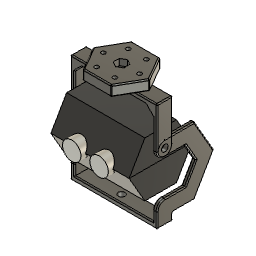
polychrome-sensor-box (Autodesk Fusion 360 design; units mm, degrees)
Autodesk Fusion 360 part; units mm, degrees
note: some values were not read from the file. Set by a fixed rule: which face or edge a step refers to.
(part 1 of 2)
sketch "base" plane through (0, 0, 0) normal (0, 0, 1) x (1, 0, 0) in component "Component"
  line L0 (31.5, 19.5) -> (-31.5, 19.5)
  line L1 (-31.5, 19.5) -> (-31.5, -19.5)
  line L2 (-31.5, -19.5) -> (31.5, -19.5)
  line L3 (31.5, -19.5) -> (31.5, 19.5)
  line L4 (31.5, 19.5) -> (-31.5, -19.5) construction
  line L5 (-31.5, 19.5) -> (31.5, -19.5) construction
  dimension "d5" = 63
  dimension "d6" = 39
  constraint horizontal L0
  constraint perpendicular L0 L1
  constraint parallel L0 L2
  constraint parallel L1 L3
  constraint coincident L4 origin
  constraint coincident L5 origin
  measures "d5" distance of L1.end L2.end
  measures "d6" distance of L0.end L1.end
extrude "Extrude1" add sketch "base" along normal blind 36 makes body 1 in component "Component"
shell "Shell1" thickness 2 removed faces 1 at (10.5, 6.5, 36) on bodies 1 in component "Component"
sketch "sensors" plane through (0, -19.5, 0) normal (0, -1, 0) x (1, 0, 0) in component "Component"
  line L0 (-31.5, 0) -> (31.5, 0)
  line L1 (31.5, 0) -> (31.5, 36)
  line L2 (31.5, 36) -> (-31.5, 36)
  line L3 (-31.5, 36) -> (-31.5, 0)
  line L4 (-31.5, 24.25) -> (31.5, 24.25) construction
  line L5 (0, 36) -> (0, 0) construction
  line L6 (6.219, 36) -> (6.219, 0) construction
  circle A0 centre (18.719, 24.25) radius 8.65
  circle A1 centre (-6.281, 24.25) radius 8.65
  dimension "d10" = 24.25
  dimension "d63" = 6.219
  dimension "d64" = 17.3
  dimension "d65" = 12.5
  constraint coincident L3 L4.start
  constraint coincident L1 L4.end
  constraint perpendicular L1 L4
  constraint midpoint L2 L5.start
  constraint coincident L5.end origin
  constraint coincident L2 L6.start
  constraint coincident L0 L6.end
  constraint perpendicular L0 L6
  constraint coincident L4 A0.centre
  constraint symmetric L6 A0 A1
  measures "d10" distance of L0 L4
  measures "d63" distance of L5 L6
  measures "d64" diameter of A0
  measures "d65" distance of L6 A0.centre
extrude "Extrude2" cut sketch "sensors" against normal up to surface (2 mm away) contours A0 | A1 bodies 1 in component "Component"
sketch "rj45" plane through (-31.5, 0, 0) normal (-1, 0, 0) x (0, -1, 0) in component "Component"
  line L0 (-19.5, 0) -> (19.5, 0)
  line L1 (19.5, 0) -> (19.5, 36)
  line L2 (19.5, 36) -> (-19.5, 36)
  line L3 (-19.5, 36) -> (-19.5, 0)
  line L4 (-4.499, 36) -> (-4.499, 0) construction
  line L5 (-19.5, 13.6) -> (19.5, 13.6) construction
  line L6 (3.901, 21) -> (-12.899, 21)
  line L7 (-12.899, 21) -> (-12.899, 6.2)
  line L8 (-12.899, 6.2) -> (3.901, 6.2)
  line L9 (3.901, 6.2) -> (3.901, 21)
  line L10 (3.901, 21) -> (-12.899, 6.2) construction
  line L11 (-12.899, 21) -> (3.901, 6.2) construction
  point P0 (-4.499, 13.6)
  dimension "d57" = 15.001
  dimension "d58" = 13.6
  dimension "d59" = 16.8
  dimension "d60" = 14.8
  constraint coincident L2 L4.start
  constraint coincident L0 L4.end
  constraint perpendicular L0 L4
  constraint coincident L3 L5.start
  constraint coincident L1 L5.end
  constraint perpendicular L1 L5
  constraint horizontal L6
  constraint perpendicular L6 L7
  constraint parallel L6 L8
  constraint parallel L7 L9
  constraint coincident L10 P0
  constraint coincident L11 P0
  constraint coincident L4 P0
  constraint coincident L5 P0
  measures "d57" distance of L3 L4
  measures "d58" distance of L0 L5
  measures "d59" distance of L7.end L8.end
  measures "d60" distance of L6.end L7.end
extrude "Extrude3" cut sketch "rj45" against normal up to surface (2 mm away) contours L6 L7 L8 L9 bodies 1 in component "Component"
sketch "Sketch2" plane through (0, 0, 0) normal (0, 0, 1) x (1, 0, 0) in component "sensor"
  line L0 (0, 0) -> (57, 0)
  line L1 (57, 0) -> (57, 30)
  line L2 (57, 30) -> (0, 30)
  line L3 (0, 30) -> (0, 0)
  dimension "d66" = 57
  dimension "d67" = 30
  constraint horizontal L0
  constraint vertical L1
  constraint horizontal L2
  constraint vertical L3
  constraint coincident L0.start L3.end
  measures "d66" distance of L0.start L0.end
  measures "d67" distance of L0.start L2.end
extrude "Extrude1'" add sketch "Sketch2" along normal blind 1.6 separate body makes body 2 in component "sensor"
sketch "Sketch3" plane through (0, 0, 1.6) normal (0, 0, 1) x (-1, 0, 0) in component "sensor"
  line L0 (0, -30) -> (0, 0)
  line L1 (0, 0) -> (-57, 0)
  line L2 (-57, 0) -> (-57, -30)
  line L3 (-57, -30) -> (0, -30)
  line L4 (-21.823, -25.799) -> (5.277, -25.799)
  line L5 (5.277, -25.799) -> (5.277, -8.999)
  line L6 (5.277, -8.999) -> (-21.823, -8.999)
  line L7 (-21.823, -8.999) -> (-21.823, -25.799)
  line L8 (-21.823, -25.799) -> (5.277, -8.999) construction
  line L9 (5.277, -25.799) -> (-21.823, -8.999) construction
  line L10 (-29.029, -6.623) -> (-40.409, -6.623)
  line L11 (-40.409, -6.623) -> (-40.409, -3.283)
  line L12 (-40.409, -3.283) -> (-29.029, -3.283)
  line L13 (-29.029, -3.283) -> (-29.029, -6.623)
  line L14 (-29.029, -6.623) -> (-40.409, -3.283) construction
  line L15 (-40.409, -6.623) -> (-29.029, -3.283) construction
  point P0 (-8.273, -17.399)
  point P1 (-8.273, -17.399)
  point P2 (-34.719, -4.953)
  point P3 (-34.719, -4.953)
  dimension "d70" = 12.601
  dimension "d71" = 8.273
  dimension "d72" = 27.1
  dimension "d73" = 16.8
  dimension "d76" = 25.047
  dimension "d77" = 34.719
  dimension "d78" = 11.38
  dimension "d79" = 3.34
  constraint horizontal L4
  constraint perpendicular L4 L5
  constraint parallel L4 L6
  constraint parallel L5 L7
  constraint coincident L8 P1
  constraint coincident L9 P1
  constraint coincident P1 P0
  constraint horizontal L10
  constraint perpendicular L10 L11
  constraint parallel L10 L12
  constraint parallel L11 L13
  constraint coincident L14 P3
  constraint coincident L15 P3
  constraint coincident P3 P2
  measures "d70" distance of L3 P1
  measures "d71" distance of L0 P1
  measures "d72" distance of L5.end L6.end
  measures "d73" distance of L4.end L5.end
  measures "d76" distance of L3 P3
  measures "d77" distance of L0 P3
  measures "d78" distance of L11.end L12.end
  measures "d79" distance of L10.end L11.end
extrude "Extrude2'" add sketch "Sketch3" along normal blind 14.8 contours L0 L4 L6 L7 | L0 L4 L5 L6 bodies 2 in component "sensor"
extrude "Extrude3'" add sketch "Sketch3" along normal blind 28.8 contours L10 L11 L12 L13 bodies 2 in component "sensor"
sketch "Sketch4" plane through (0, 3.283, 0) normal (0, -1, 0) x (1, 0, 0) in component "sensor"
  line L0 (29.029, 1.6) -> (40.409, 1.6)
  line L1 (40.409, 1.6) -> (40.409, 30.4)
  line L2 (40.409, 30.4) -> (29.029, 30.4)
  line L3 (29.029, 30.4) -> (29.029, 1.6)
  line L4 (29.029, 30.4) -> (40.2114, 30.4)
  line L5 (40.2114, 30.4) -> (40.2114, 9.1)
  line L6 (40.2114, 9.1) -> (29.029, 9.1)
  line L7 (29.029, 9.1) -> (29.029, 30.4)
  dimension "d82" = 21.3
  constraint horizontal L4
  constraint vertical L5
  constraint horizontal L6
  constraint vertical L7
  constraint coincident L2.end L3.start
  measures "d82" distance of L2.end L6.end
extrude "Extrude4" add sketch "Sketch4" along normal blind 8 separate body contours L2 L3 L4 L5 L6 L7 makes body 3 in component "sensor"
ref_plane "WorkPlane1" through (34.6202, -0.717, 19.75) normal (1, 0, 0) x (0, 0, 1) in component "sensor"
ref_plane "WorkPlane2" through (57.7702, -0.717, 19.75) normal (1, 0, 0) x (0, 0, 1) in component "sensor"
ref_plane "WorkPlane3" through (11.4702, -0.717, 19.75) normal (1, 0, 0) x (0, 0, 1) in component "sensor"
extrude "Extrude5" add 1 faces at (40.2114, -2.0503, 16.2) along direction (1, 0, 0) up to surface (17.5588 mm away) and the other way up to surface (28.7412 mm away) on bodies 3 bodies 2 3 in component "sensor"
sketch "Sketch5" plane through (0, -4.717, 0) normal (0, -1, 0) x (1, 0, 0) in component "sensor"
  line L0 (11.4702, 9.1) -> (57.7702, 9.1)
  line L1 (57.7702, 9.1) -> (57.7702, 30.4)
  line L2 (57.7702, 30.4) -> (11.4702, 30.4)
  line L3 (11.4702, 30.4) -> (11.4702, 9.1)
  line L4 (11.4702, 19.75) -> (57.7702, 19.75) construction
  line L5 (34.6202, 30.4) -> (34.6202, 9.1) construction
  circle A0 centre (21.4702, 19.75) radius 8.9
  circle A1 centre (47.7702, 19.75) radius 8.9
  dimension "d91" = 17.8
  dimension "d92" = 10
  constraint midpoint L3 L4.start
  constraint midpoint L1 L4.end
  constraint midpoint L2 L5.start
  constraint midpoint L0 L5.end
  constraint coincident L4 A0.centre
  constraint symmetric L5 A0 A1
  measures "d91" diameter of A0
  measures "d92" distance of L4.start A0.centre
extrude "Extrude6" add sketch "Sketch5" along normal blind 15 contours A0 | A1 bodies 2 in component "sensor"
sketch "Sketch2 (2)" plane through (56.4993, 0, 0) normal (1, 0, 0) x (0, 1, 0) in component "Component'"
  line L0 (-8.1168, 6.6878) -> (-0.1168, 6.6878)
  line L1 (-0.1168, 6.6878) -> (-0.1168, 27.9878)
  line L2 (-0.1168, 27.9878) -> (-8.1168, 27.9878)
  line L3 (-8.1168, 27.9878) -> (-8.1168, 6.6878)
  line L4 (-8.1168, 27.9878) -> (26.6636, -2.3727) construction
  line L5 (-8.8786, 28.508) -> (-13.3996, 4.9377)
  line L6 (-13.3996, 4.9377) -> (4.7524, -10.7628)
  line L7 (4.7524, -10.7628) -> (27.4254, -2.893)
  line L8 (27.4254, -2.893) -> (31.9464, 20.6774)
  line L9 (31.9464, 20.6774) -> (13.7944, 36.3779)
  line L10 (13.7944, 36.3779) -> (-8.8786, 28.508)
  line L11 (-15.5813, 4.1804) -> (4.3173, -13.0308)
  line L12 (4.3173, -13.0308) -> (29.1721, -4.4037)
  line L13 (29.1721, -4.4037) -> (34.1281, 21.4346)
  line L14 (34.1281, 21.4346) -> (14.2295, 38.6459)
  line L15 (14.2295, 38.6459) -> (-10.6253, 30.0188)
  line L16 (-10.6253, 30.0188) -> (-15.5813, 4.1804)
  point P0 (9.2734, 12.8075)
  dimension "d96" = 24
  dimension "d104" = 2
  constraint coincident L2.end L3.start
  constraint midpoint L4 P0
  measures "d96" distance of L5.start P0
ref_plane "WorkPlane4" through (34.6202, 0.953, 19.75) normal (0, 0, 1) x (1, 0, 0) in component "sensor"
sketch "Sketch3 (2)" plane through (56.4993, 0, 0) normal (1, 0, 0) x (0, 1, 0) in component "Component'"
  line L0 (38.5849, 17.0433) -> (25.1323, 40.4534)
  line L1 (25.1323, 40.4534) -> (-1.8676, 40.5081)
  line L2 (-1.8676, 40.5081) -> (-15.415, 17.1529)
  line L3 (-15.415, 17.1529) -> (-1.9625, -6.2572)
  line L4 (-1.9625, -6.2572) -> (25.0375, -6.3119)
  line L5 (25.0375, -6.3119) -> (38.5849, 17.0433)
  line L6 (-3.1212, -8.2548) -> (26.1881, -8.3143)
  line L7 (26.1881, -8.3143) -> (40.8943, 17.0387)
  line L8 (40.8943, 17.0387) -> (26.2911, 42.451)
  line L9 (26.2911, 42.451) -> (-3.0183, 42.5105)
  line L10 (-3.0183, 42.5105) -> (-17.7244, 17.1576)
  line L11 (-17.7244, 17.1576) -> (-3.1212, -8.2548)
  point P0 (11.5849, 17.0981)
  dimension "d111" = 27
  dimension "d112" = 2
  measures "d111" distance of L0.start P0
sketch "inner base" plane through (0, 0, 2) normal (0, 0, 1) x (-1, 0, 0) in component "Component"
  line L0 (-29.5, 17.5) -> (-29.5, -17.5)
  line L1 (-29.5, -17.5) -> (29.5, -17.5)
  line L2 (29.5, -17.5) -> (29.5, 17.5)
  line L3 (29.5, 17.5) -> (-29.5, 17.5)
  line L4 (29.5, -17.5) -> (9.5, -17.5)
  line L5 (9.5, -17.5) -> (9.5, -14)
  line L6 (9.5, -14) -> (29.5, -14)
  line L7 (29.5, -14) -> (29.5, -17.5)
  line L8 (29.5, -17.5) -> (26, -17.5)
  line L9 (26, -17.5) -> (26, 5.9)
  line L10 (26, 5.9) -> (29.5, 5.9)
  line L11 (29.5, 5.9) -> (29.5, -17.5)
  line L12 (-29.5, -17.5) -> (-29.5, 17.5) construction
  line L13 (26.5811, 12.7) -> (-29.5, 12.7) construction
  line L14 (-29.5, -17.5) -> (-19.5, -17.5)
  line L15 (-19.5, -17.5) -> (-19.5, 17.5)
  line L16 (-19.5, 17.5) -> (-29.5, 17.5)
  line L17 (-29.5, 17.5) -> (-29.5, -17.5)
  line L18 (29.5, 5.9) -> (19.5, 5.9)
  line L19 (19.5, 5.9) -> (19.5, 17.5)
  line L20 (19.5, 17.5) -> (29.5, 17.5)
  line L21 (29.5, 17.5) -> (29.5, 5.9)
  dimension "d31" = 20
  dimension "d32" = 3.5
  dimension "d33" = 3.5
  dimension "d34" = 23.4
  dimension "d36" = 7.4
  dimension "d37" = 59
  dimension "d38" = 10
  dimension "d40" = 10
  constraint horizontal L4
  constraint vertical L5
  constraint horizontal L6
  constraint vertical L7
  constraint coincident L1.end L2.start
  constraint horizontal L8
  constraint vertical L9
  constraint horizontal L10
  constraint vertical L11
  constraint coincident L1 L0.end
  constraint coincident L3 L0.start
  constraint perpendicular L3 L12
  constraint coincident L12 L13.end
  constraint perpendicular L12 L13
  constraint horizontal L14
  constraint vertical L15
  constraint horizontal L16
  constraint vertical L17
  constraint horizontal L18
  constraint vertical L19
  constraint horizontal L20
  constraint vertical L21
  measures "d31" distance of L1.end L4.end
  measures "d32" distance of L1.end L6.end
  measures "d33" distance of L1.end L8.end
  measures "d34" distance of L1.end L10.end
  measures "d36" distance of L10.end L13.start
  measures "d37" distance of L2 L12
  measures "d38" distance of L0.end L14.end
  measures "d40" distance of L10.end L18.end
extrude "Extrude4'" add sketch "inner base" along normal blind 3 contours L0 L1 L3 L14 L15 L16 L17 | L2 L3 L10 L18 L19 L20 L21 | L1 L4 L5 L6 L9 | L1 L2 L4 L6 L7 L8 L9 L11 | L2 L6 L9 L10 L11 L18 bodies 1 in component "Component"
sketch "board holes" plane through (0, 0, 5) normal (0, 0, 1) x (-1, 0, 0) in component "Component"
  line L0 (29.5, 17.5) -> (19.5, 17.5)
  line L1 (19.5, 17.5) -> (19.5, 5.9)
  line L2 (19.5, 5.9) -> (26, 5.9)
  line L3 (26, 5.9) -> (26, -14)
  line L4 (26, -14) -> (9.5, -14)
  line L5 (9.5, -14) -> (9.5, -17.5)
  line L6 (9.5, -17.5) -> (29.5, -17.5)
  line L7 (29.5, -17.5) -> (29.5, 17.5)
  line L8 (29.1, -17.1) -> (-27.9, -17.1) construction
  line L9 (-27.9, -17.1) -> (-27.9, 12.9) construction
  line L10 (-27.9, 12.9) -> (29.1, 12.9) construction
  line L11 (29.1, 12.9) -> (29.1, -17.1) construction
  line L12 (26.893, -17.1) -> (26.893, 12.9) construction
  line L13 (29.1, -15.04) -> (-27.9, -15.04) construction
  line L14 (29.1, 10.614) -> (-27.9, 10.614) construction
  circle A0 centre (26.893, -15.04) radius 1.25
  circle A1 centre (26.893, 10.614) radius 1.25
  line L15 (-25.9, -17.1) -> (-25.9, 12.9) construction
  circle A2 centre (-25.9, -15.04) radius 1.25
  circle A3 centre (-25.9, 10.614) radius 1.25
  dimension "d43" = 57
  dimension "d44" = 30
  dimension "d45" = 0.4
  dimension "d46" = 0.4
  dimension "d47" = 2.207
  dimension "d48" = 2.06
  dimension "d49" = 2.286
  dimension "d50" = 2.5
  dimension "d51" = 2.5
  dimension "d52" = 52.793
  dimension "d53" = 2.5
  dimension "d54" = 2.5
  constraint horizontal L8
  constraint vertical L9
  constraint horizontal L10
  constraint vertical L11
  constraint coincident L8 L12.start
  constraint coincident L10 L12.end
  constraint perpendicular L10 L12
  constraint coincident L11 L13.start
  constraint coincident L9 L13.end
  constraint perpendicular L9 L13
  constraint coincident L11 L14.start
  constraint coincident L9 L14.end
  constraint perpendicular L9 L14
  constraint coincident L12 A0.centre
  constraint coincident L13 A0.centre
  constraint coincident L12 A1.centre
  constraint coincident L14 A1.centre
  constraint coincident L8 L15.start
  constraint coincident L10 L15.end
  constraint perpendicular L10 L15
  constraint coincident L13 A2.centre
  constraint coincident L15 A2.centre
  constraint coincident L14 A3.centre
  constraint coincident L15 A3.centre
  measures "d43" distance of L8.start L8.end
  measures "d44" distance of L8.start L10.end
  measures "d45" distance of L6 L8
  measures "d46" distance of L7 L11
  measures "d47" distance of L11 L12
  measures "d48" distance of L8 L13
  measures "d49" distance of L10 L14
  measures "d50" diameter of A0
  measures "d51" diameter of A1
  measures "d52" distance of L12 L15
  measures "d53" diameter of A2
  measures "d54" diameter of A3
extrude "Extrude5'" cut sketch "board holes" against normal blind 4 draft -8 contours A0 | A1 | A2 | A3 bodies 1 in component "Component"
sketch "Sketch6" plane through (31.5, 0, 0) normal (1, 0, 0) x (0, 1, 0) in component "Component"
  line L0 (-19.5, 0) -> (19.5, 0)
  line L1 (19.5, 0) -> (19.5, 36)
  line L2 (19.5, 36) -> (-19.5, 36)
  line L3 (-19.5, 36) -> (-19.5, 0)
  line L4 (-19.5, 36) -> (19.5, 0) construction
  line L5 (19.5, 36) -> (-19.5, 0) construction
  constraint coincident L2.end L3.start
  constraint coincident L0.end L1.start
  constraint coincident L1.end L2.start
  constraint coincident L0.start L3.end
extrude "Extrude6'" add sketch "Sketch3 (2)" along normal blind 2 separate body contours L0 L1 L2 L3 L4 L5 makes body 4 in component "Component'"
extrude "Extrude7" add sketch "Sketch3 (2)" along normal blind 2 and the other way up to surface (57.7702 mm away) bodies 4 in component "Component'"
sketch "Sketch6 (2)" plane through (0, 0, 0) normal (0, 0, -1) x (1, 0, 0) in component "sensor"
  line L0 (0, 0) -> (0, -30)
  line L1 (0, -30) -> (57, -30)
  line L2 (57, -30) -> (57, 0)
  line L3 (57, 0) -> (0, 0)
  line L4 (0, -2.286) -> (56.7828, -2.286) construction
  line L5 (0, -27.94) -> (57, -27.94) construction
  line L6 (2.207, 0) -> (2.207, -30) construction
  line L7 (55, 0) -> (55, -30) construction
  circle A0 centre (55, -2.4077) radius 1.262
  circle A1 centre (55, -27.94) radius 1.262
  circle A2 centre (2.207, -27.94) radius 1.262
  circle A3 centre (2.207, -2.286) radius 1.262
  line L8 (6.5, 0) -> (47, 0)
  line L9 (47, 0) -> (47, -30)
  line L10 (47, -30) -> (6.5, -30)
  line L11 (6.5, -30) -> (6.5, 0)
  line L12 (47, -10) -> (57, -10)
  line L13 (57, -10) -> (57, -20)
  line L14 (57, -20) -> (47, -20)
  line L15 (47, -20) -> (47, -10)
  line L16 (0, -6.5) -> (6.5, -6.5)
  line L17 (6.5, -6.5) -> (6.5, -27.5)
  line L18 (6.5, -27.5) -> (0, -27.5)
  line L19 (0, -27.5) -> (0, -6.5)
  dimension "d119" = 2.286
  dimension "d120" = 2.207
  dimension "d121" = 2.06
  dimension "d122" = 2
  dimension "d123" = 2.524
  dimension "d124" = 2.524
  dimension "d125" = 2.524
  dimension "d126" = 2.524
  dimension "d131" = 6.5
  dimension "d132" = 10
  dimension "d133" = 10
  dimension "d134" = 10
  dimension "d135" = 6.5
  dimension "d136" = 2.5
  constraint coincident L0 L4.start
  constraint perpendicular L2 L4
  constraint coincident L0 L5.start
  constraint coincident L2 L5.end
  constraint perpendicular L2 L5
  constraint coincident L3 L6.start
  constraint coincident L1 L6.end
  constraint perpendicular L1 L6
  constraint coincident L3 L7.start
  constraint coincident L1 L7.end
  constraint perpendicular L1 L7
  constraint coincident L7 A0.centre
  constraint coincident L5 A1.centre
  constraint coincident L7 A1.centre
  constraint coincident L6 A2.centre
  constraint coincident L5 A2.centre
  constraint coincident L4 A3.centre
  constraint coincident L6 A3.centre
  constraint horizontal L8
  constraint vertical L9
  constraint horizontal L10
  constraint vertical L11
  constraint coincident L1 L9.end
  constraint coincident L3 L8.start
  constraint horizontal L12
  constraint vertical L13
  constraint horizontal L14
  constraint vertical L15
  constraint coincident L2 L13.end
  constraint coincident L9 L12.start
  constraint horizontal L16
  constraint vertical L17
  constraint horizontal L18
  constraint vertical L19
  constraint coincident L11 L17.end
  constraint coincident L0 L16.start
  measures "d119" distance of L3 L4
  measures "d120" distance of L0 L6
  measures "d121" distance of L1 L5
  measures "d122" distance of L2 L7
  measures "d123" diameter of A0
  measures "d124" diameter of A1
  measures "d125" diameter of A2
  measures "d126" diameter of A3
  measures "d131" distance of L0 L11
  measures "d132" distance of L2 L9
  measures "d133" distance of L3 L12
  measures "d134" distance of L1 L14
  measures "d135" distance of L3 L16
  measures "d136" distance of L1 L18
extrude "Extrude7'" add sketch "Sketch6 (2)" along normal blind 2 contours L0 A2 L11 L16 L17 L18 L19 | L1 L3 L8 L9 L10 L11 L15 L17 | A2 L18 | L2 L9 L12 L13 L14 L15 picked at (2.177, -27.2271) bodies 2 in component "sensor"
extrude "Extrude8" add sketch "Sketch6 (2)" along normal blind 4 draft -8 contours A2 L18 | A2 L18 | A0 | A1 | A3 bodies 2 in component "sensor"
ref_plane "WorkPlane5" through (34.6202, -4.717, 19.75) normal (1, 0, 0) x (0, 0, -1) in component "sensor"
ref_plane "WorkPlane4" through (0.8755, 14.3886, 3.4379) normal (-1, 0, 0) x (0, -1, 0) in component "enclosure"
sketch "Sketch3 (3)" plane through (0.8755, 0, 0) normal (-1, 0, 0) x (0, -1, 0) in component "enclosure"
  line L0 (-29.3886, 3.6379) -> (0.6114, 3.6379) construction
  line L1 (5.3284, 34.0379) -> (5.3284, 12.7379) construction
  line L2 (5.3284, 23.3879) -> (-27.8442, 23.3879) construction
  line L3 (-14.3886, 3.6379) -> (-14.3886, 31.9391) construction
  line L4 (-0.3886, -0.8608) -> (13.6114, 23.3879)
  line L5 (13.6114, 23.3879) -> (-0.3886, 47.6367)
  line L6 (-0.3886, 47.6367) -> (-28.3886, 47.6367)
  line L7 (-28.3886, 47.6367) -> (-42.3886, 23.3879)
  line L8 (-42.3886, 23.3879) -> (-28.3886, -0.8608)
  line L9 (-28.3886, -0.8608) -> (-0.3886, -0.8608)
  line L10 (-5.8886, 1.6379) -> (-26.8886, 1.6379)
  line L11 (-44.698, 23.3879) -> (-29.5433, -2.8608)
  line L12 (-29.5433, -2.8608) -> (0.7661, -2.8608)
  line L13 (0.7661, -2.8608) -> (15.9208, 23.3879)
  line L14 (15.9208, 23.3879) -> (0.7661, 49.6367)
  line L15 (0.7661, 49.6367) -> (-29.5433, 49.6367)
  line L16 (-29.5433, 49.6367) -> (-44.698, 23.3879)
  point P0 (5.3284, 34.0379)
  point P1 (5.3284, 12.7379)
  point P2 (0.6114, 3.6379)
  point P3 (-29.3886, 3.6379)
  point P4 (-14.3886, 23.3879)
  dimension "d156" = 28
  dimension "d157" = 2
  constraint coincident P3 L0.start
  constraint coincident P2 L0.end
  constraint coincident P0 L1.start
  constraint coincident P1 L1.end
  constraint midpoint L1 L2.start
  constraint perpendicular L1 L2
  constraint midpoint L0 L3.start
  constraint perpendicular L0 L3
  constraint coincident L2 P4
  constraint coincident L3 P4
  constraint parallel L9 L10
  measures "d156" distance of L4.start P4
extrude "Extrude4''" add sketch "Sketch3 (3)" along normal blind 2 separate body contours L4 L5 L6 L7 L8 L9 makes body 5 in component "enclosure"
mirror "Mirror1" about plane through (36.4957, -5.3284, 23.3879) normal (1, 0, 0) of bodies 5 makes body 6 in component "enclosure"
extrude "Extrude5''" add sketch "Sketch3 (3)" along normal blind 2 and the other way up to surface (73.2404 mm away) separate body makes body 7 in component "enclosure"
extrude "Extrude6''" add 1 faces at (49.0357, 19.0552, -0.8608) along direction (0, 0, 1) up to surface (4.4987 mm away) on bodies 7 bodies 7 in component "enclosure"
extrude "Extrude7''" add 1 faces at (49.0357, 0.3886, 2.1384) along direction (0, -1, 0) up to surface end surface through (0.8755, 0.3886, -0.8608) normal (0, 0.866025, 0.5) offset 0 on bodies 7 bodies 7 in component "enclosure"
extrude "Extrude8'" add 1 faces at (23.9556, 28.3886, 0.6388) along direction (0, 1, 0) up to surface end surface through (0.8755, 42.3886, 23.3879) normal (0, -0.866025, 0.5) offset 0 on bodies 7 bodies 7 in component "enclosure"
ref_plane "WorkPlane5" through (36.4957, 14.3886, 23.3879) normal (0, 0, 1) x (0, 1, 0) in component "enclosure"
split "Split1" by plane through (36.4957, 14.3886, 23.3879) normal (0, 0, 1) bodies 7 makes body 8 at (49.0357, -10.8693, 32.1375) in component "enclosure"
sketch "Sketch4 (2)" plane through (-1.1245, 0, 0) normal (-1, 0, 0) x (0, -1, 0) in component "enclosure"
  line L0 (15.9208, 23.3879) -> (13.6114, 23.3879)
  line L1 (13.6114, 23.3879) -> (2.2088, 3.6379)
  line L2 (2.2088, 3.6379) -> (-30.9859, 3.6379)
  line L3 (-30.9859, 3.6379) -> (-42.3886, 23.3879)
  line L4 (-42.3886, 23.3879) -> (-44.698, 23.3879)
  line L5 (-44.698, 23.3879) -> (-29.5433, -2.8608)
  line L6 (-29.5433, -2.8608) -> (0.7661, -2.8608)
  line L7 (0.7661, -2.8608) -> (15.9208, 23.3879)
  line L8 (13.6114, 23.3879) -> (11.6114, 23.3879)
  line L9 (11.6114, 23.3879) -> (9.6114, 19.9238)
  line L10 (9.6114, 19.9238) -> (11.1114, 19.0578)
  line L11 (9.6114, 16.4597) -> (6.1473, 18.4597) construction
  line L12 (6.1473, 18.4597) -> (11.302, 27.3879)
  line L13 (-0.3886, 47.6367) -> (13.6114, 23.3879)
  line L14 (8.9188, 19.1242) -> (11.9006, 24.2889) construction
  line L15 (13.0993, 17.6792) -> (7.5473, 20.8846) construction
  line L16 (9.3382, 19.8506) -> (11.0114, 18.8846)
  line L17 (11.6114, 23.3879) -> (10.186, 23.3879) construction
  line L18 (9.3382, 19.8506) -> (11.3805, 23.3879)
  line L19 (11.6114, 23.3879) -> (11.3805, 23.3879)
  line L20 (7.5473, 20.8846) -> (7.5473, 11.8372) construction
  line L21 (7.5473, 20.8846) -> (7.5473, 12.8846)
  dimension "d172" = 2
  dimension "d173" = 4
  dimension "d174" = 3
  dimension "d175" = 4
  dimension "d177" = 0.2
  dimension "d178" = 0.2
  constraint coincident L0.end L1.start
  constraint parallel L0 L8
  constraint parallel L1 L9
  constraint coincident L1 L10.end
  constraint perpendicular L1 L10
  constraint coincident L1 L11.start
  constraint parallel L10 L11
  constraint coincident L11 L12.start
  constraint coincident L12.end L13
  constraint parallel L9 L12
  constraint parallel L9 L14
  constraint parallel L10 L15
  constraint coincident L15 L16.start
  constraint coincident L14 L16.start
  constraint coincident L15 L16.end
  constraint coincident L1 L16.end
  constraint parallel L8 L17
  constraint coincident L14 L18.end
  constraint coincident L17 L18.end
  constraint perpendicular L2 L20
  constraint coincident L12 L15.end
  constraint coincident L15.end L20
  constraint coincident L15.end L20.start
  constraint coincident L1 L21.end
  constraint coincident L20 L21.end
  constraint coincident L11.end L12.start
  measures "d172" distance of L0.end L8.end
  measures "d173" distance of L8.end L9.end
  measures "d174" distance of L10.end L11.start
  measures "d175" distance of L11.start L11.end
  measures "d177" distance of L9 L14
  measures "d178" distance of L10 L15
extrude "Extrude9" add sketch "Sketch4 (2)" against normal blind 14.4 separate body contours L1 L8 L9 L10 makes body 9 in component "enclosure"
extrude "Extrude10" cut 1 faces at (-1.1245, -12.1114, 21.9446) along direction (1, 0, 0) blind 5.4 on bodies 9 bodies 9 in component "enclosure"
mirror "Mirror2" about plane through (36.4957, -5.3284, 23.3879) normal (1, 0, 0) of bodies 9 makes body 10 in component "enclosure"
extrude "Extrude11" add sketch "Sketch4 (2)" against normal blind 14.4 separate body contours L1 L8 L12 L13 L16 L18 L19 L21 makes body 11 in component "enclosure"
extrude "Extrude12" cut sketch "Sketch4 (2)" against normal blind 5.4 contours L1 L8 L12 L13 L16 L18 L19 L21 bodies 11 in component "enclosure"
mirror "Mirror3" about plane through (36.4957, -5.3284, 23.3879) normal (1, 0, 0) of bodies 11 makes body 12 in component "enclosure"
sketch "Sketch5 (2)" plane through (0, 0, 23.3879) normal (0, 0, 1) x (1, 0, 0) in component "enclosure"
  line L0 (-1.1245, 42.3886) -> (74.1158, 42.3886) construction
  line L1 (36.4957, 42.3886) -> (36.4957, 32.3886) construction
  line L2 (41.4957, 42.3886) -> (31.4957, 42.3886)
  line L3 (31.4957, 42.3886) -> (31.4957, 32.3886)
  line L4 (31.4957, 32.3886) -> (41.4957, 32.3886)
  line L5 (41.4957, 32.3886) -> (41.4957, 42.3886)
  line L6 (41.4957, 42.3886) -> (31.4957, 32.3886) construction
  line L7 (31.4957, 42.3886) -> (41.4957, 32.3886) construction
  circle A0 centre (36.4957, 37.3886) radius 1.45
  point P0 (-1.1245, 42.3886)
  point P1 (74.1158, 42.3886)
  point P2 (36.4957, 37.3886)
  dimension "d191" = 10
  dimension "d192" = 10
  dimension "d193" = 10
  dimension "d198" = 2.9
  constraint coincident P0 L0.start
  constraint coincident P1 L0.end
  constraint midpoint L0 L1.start
  constraint perpendicular L0 L1
  constraint horizontal L2
  constraint perpendicular L2 L3
  constraint parallel L2 L4
  constraint parallel L3 L5
  constraint coincident L6 P2
  constraint coincident L7 P2
  constraint midpoint L1 P2
  constraint coincident P2 A0.centre
  measures "d191" distance of L1.start L1.end
  measures "d192" distance of L3.end L4.end
  measures "d193" distance of L2.end L3.end
  measures "d198" diameter of A0
extrude "Extrude13" add sketch "Sketch5 (2)" along normal up to surface contours L2 L3 L4 L5 | A0 end surface through (0.8755, 42.3886, 23.3879) normal (0, -0.866025, 0.5) offset 0 bodies 7 in component "enclosure"
extrude "Extrude14" add sketch "Sketch5 (2)" along normal up to surface contours L2 L3 L4 L5 | A0 end surface through (0.8755, 28.3886, 47.6367) normal (0, -0.866025, -0.5) offset 0 bodies 8 in component "enclosure"
extrude "Extrude15" cut sketch "Sketch5 (2)" against normal blind 4 draft -8 contours A0 bodies 7 in component "enclosure"
extrude "Extrude16" cut sketch "Sketch5 (2)" along normal up to surface contours A0 end surface through (0.8755, 29.5433, 49.6367) normal (0, 0.866025, 0.5) offset 0 bodies 8 in component "enclosure"
ref_plane "WorkPlane6" through (36.4957, 14.3886, 25.3879) normal (0, 0, 1) x (0, 1, 0) in component "enclosure"
sketch "Sketch6 (3)" plane through (0, 0, 25.3879) normal (0, 0, 1) x (1, 0, 0) in component "enclosure"
  circle A0 centre (36.4957, 37.3886) radius 3
  point P0 (36.4957, 37.3886)
  dimension "d204" = 6
  constraint coincident P0 A0.centre
  measures "d204" diameter of A0
extrude "Extrude17" cut sketch "Sketch6 (3)" along normal up to surface end surface through (0.8755, 29.5433, 49.6367) normal (0, 0.866025, 0.5) offset 0 bodies 8 in component "enclosure"
combine "Combine1" operation add target body 12 tool bodies 8 11 in component "enclosure"
combine "Combine2" operation add target body 7 tool bodies 10 9 in component "enclosure"
split "Split2" by plane through (36.4957, 14.3886, 23.3879) normal (0, 0, 1) bodies 6 makes body 13 at (74.1158, 19.0552, 31.4708) in component "enclosure"
split "Split3" by plane through (36.4957, 14.3886, 23.3879) normal (0, 0, 1) bodies 5 makes body 14 at (0.8755, 19.0552, 31.4708) in component "enclosure"
combine "Combine3" operation add target body 7 tool bodies 6 5 in component "enclosure"
combine "Combine4" operation add target body 12 tool bodies 13 14 in component "enclosure"
combine "Combine5" operation cut target body 7 tool bodies 2 body 2 seen with x (1, 0, 0) y (0, 1, 0) z (0, 0, 1) at (1.8755, -0.6114, 3.6379) keep tools in component "enclosure"
combine "Combine6" operation cut target body 12 tool bodies 2 body 2 seen with x (1, 0, 0) y (0, 1, 0) z (0, 0, 1) at (1.8755, -0.6114, 3.6379) keep tools in component "enclosure"
sketch "Sketch7" plane through (72.1158, 0, 0) normal (-1, 0, 0) x (0, -1, 0) in component "enclosure"
  line L0 (-42.3886, 23.3879) -> (13.6114, 23.3879)
  line L1 (13.6114, 23.3879) -> (-0.3886, 47.6367)
  line L2 (-0.3886, 47.6367) -> (-28.3886, 47.6367)
  line L3 (-28.3886, 47.6367) -> (-42.3886, 23.3879)
  line L4 (-14.3886, 47.6367) -> (-14.3886, 23.3879) construction
  circle A0 centre (-14.3886, 35.5123) radius 6.5
  circle A1 centre (-14.3886, 35.5123) radius 3.2
  dimension "d207" = 13
  dimension "d214" = 6.4
  constraint midpoint L2 L4.start
  constraint midpoint L0 L4.end
  constraint midpoint L4 A0.centre
  constraint concentric A0 A1
  measures "d207" diameter of A0
  measures "d214" diameter of A1
extrude "Extrude18" add sketch "Sketch7" along normal blind 5 contours A0 | A1 bodies 12 in component "enclosure"
chamfer "Chamfer1" distance 5 angle 45 1 edges at (72.1158, 20.4487, 37.8628) on bodies 12 in component "enclosure"
sketch "Sketch8" plane through (67.1158, 0, 0) normal (-1, 0, 0) x (0, -1, 0) in component "enclosure"
  circle A0 centre (-14.3886, 35.5123) radius 6.5
  line L0 (-14.3886, 35.5123) -> (-7.8886, 35.5123) construction
  line L1 (-8.0089, 35.5123) -> (-11.1987, 41.0373)
  line L2 (-11.1987, 41.0373) -> (-17.5784, 41.0373)
  line L3 (-17.5784, 41.0373) -> (-20.7683, 35.5123)
  line L4 (-20.7683, 35.5123) -> (-17.5784, 29.9873)
  line L5 (-17.5784, 29.9873) -> (-11.1987, 29.9873)
  line L6 (-11.1987, 29.9873) -> (-8.0089, 35.5123)
  point P0 (-14.3886, 35.5123)
  dimension "d211" = 5.525
  constraint coincident P0 A0.centre
  constraint coincident A0 L0.end
  constraint horizontal L0
  constraint parallel L0 L5
  measures "d211" distance of P0 L6
extrude "Extrude19" cut sketch "Sketch8" against normal blind 5 contours L1 L2 L3 L4 L5 L6 bodies 12 in component "enclosure"
extrude "Extrude20" cut sketch "Sketch7" against normal up to surface (2 mm away) contours A1 bodies 12 in component "enclosure"
sketch "Sketch9" plane through (0.8755, 0, 0) normal (1, 0, 0) x (0, 1, 0) in component "enclosure"
  line L0 (25.1876, 20.0379) -> (25.1876, 5.2379)
  line L1 (25.1876, 5.2379) -> (8.3876, 5.2379)
  line L2 (8.3876, 5.2379) -> (8.3876, 20.0379)
  line L3 (8.3876, 20.0379) -> (25.1876, 20.0379)
  line L4 (-2.2088, 3.6379) -> (30.9859, 3.6379)
  line L5 (30.9859, 3.6379) -> (42.3886, 23.3879)
  line L6 (42.3886, 23.3879) -> (-13.6114, 23.3879)
  line L7 (-13.6114, 23.3879) -> (-2.2088, 3.6379)
  line L8 (27.3886, 23.3879) -> (37.3886, 23.3879)
  line L9 (37.3886, 23.3879) -> (37.3886, 16.3879)
  line L10 (37.3886, 16.3879) -> (27.3886, 16.3879)
  line L11 (27.3886, 16.3879) -> (27.3886, 23.3879)
  dimension "d217" = 10
  dimension "d218" = 7
  dimension "d219" = 5
  constraint horizontal L8
  constraint vertical L9
  constraint horizontal L10
  constraint vertical L11
  constraint coincident L6 L8.start
  measures "d217" distance of L8.start L8.end
  measures "d218" distance of L8.start L10.end
  measures "d219" distance of L5.end L8.end
extrude "Extrude21" add sketch "Sketch9" along normal blind 3 separate body contours L6 L8 L9 L10 L11 makes body 15 in component "enclosure"
chamfer "Chamfer2" distance 3 angle 45 1 edges at (3.8755, 32.3886, 16.3879) on bodies 15 in component "enclosure"
extrude "Extrude22" add 1 faces at (2.8755, 34.0552, 23.3879) along direction (0, 0, 1) blind 2 separate body on bodies 15 makes body 16 in component "enclosure"
extrude "Extrude23" add 1 faces at (2.8755, 34.0552, 25.3879) along direction (0, 0, 1) blind 3 draft -8 on bodies 16 bodies 7 15 16 in component "enclosure"
combine "Combine7" operation add target body 16 tool bodies 15 in component "enclosure"
ref_plane "WorkPlane7" through (-0.1245, 16.7876, 12.6379) normal (0, -1, 0) x (1, 0, 0) in component "enclosure"
mirror "Mirror4" about plane through (-0.1245, 16.7876, 12.6379) normal (0, -1, 0) of bodies 16 makes body 17 in component "enclosure"
mirror "Mirror5" about plane through (36.4957, -5.3284, 23.3879) normal (1, 0, 0) of bodies 17 16 makes body 18 at (72.1158, 34.0552, 22.3879) makes body 19 at (72.1158, 2.8532, 19.3879) in component "enclosure"
combine "Combine8" operation add target body 7 tool bodies 19 18 17 16 in component "enclosure"
sketch "Sketch10" plane through (-1.1245, 0, 0) normal (-1, 0, 0) x (0, -1, 0) in component "enclosure"
  line L0 (-44.698, 23.3879) -> (15.9208, 23.3879)
  line L1 (15.9208, 23.3879) -> (0.7661, 49.6367)
  line L2 (0.7661, 49.6367) -> (-29.5433, 49.6367)
  line L3 (-29.5433, 49.6367) -> (-44.698, 23.3879)
  circle A0 centre (-14.3886, 35.5123) radius 3.2
  point P0 (-14.3886, 35.5123)
  dimension "d233" = 6.4
  constraint coincident P0 A0.centre
  measures "d233" diameter of A0
extrude "Extrude25" cut sketch "Sketch10" against normal up to surface (2 mm away) contours A0 bodies 12 in component "enclosure"
chamfer "Chamfer3" distance 1.4 angle 45 1 edges at (33.6987, 36.3037, 25.3879) on bodies 12 in component "enclosure"
sketch "Sketch1" plane through (-1.1245, 0, 0) normal (-1, 0, 0) x (0, -1, 0) in component "holder"
  circle A0 centre (-14.3886, 35.5123) radius 3
  circle A1 centre (-14.3886, 35.5123) radius 7.5
  line L0 (-21.8886, 35.5123) -> (-6.8886, 35.5123)
  line L1 (0.7661, 49.6367) -> (-29.5433, 49.6367)
  line L2 (-44.698, 23.3879) -> (15.9208, 23.3879)
  line L3 (-42.0281, 28.0123) -> (13.251, 28.0123) construction
  line L4 (-29.5433, 49.6367) -> (-44.698, 23.3879) construction
  line L5 (15.9208, 23.3879) -> (0.7661, 49.6367) construction
  line L6 (-14.3886, 28.0123) -> (-14.3886, 4.0123) construction
  line L7 (-0.5322, 16.0123) -> (-7.4604, 28.0123)
  line L8 (-7.4604, 28.0123) -> (-21.3168, 28.0123)
  line L9 (-21.3168, 28.0123) -> (-28.245, 16.0123)
  line L10 (-28.245, 16.0123) -> (-21.3168, 4.0123)
  line L11 (-21.3168, 4.0123) -> (-7.4604, 4.0123)
  line L12 (-7.4604, 4.0123) -> (-0.5322, 16.0123)
  line L13 (1.1999, -10.9877) -> (16.7883, 16.0123)
  line L14 (16.7883, 16.0123) -> (1.1999, 43.0123)
  line L15 (1.1999, 43.0123) -> (-29.977, 43.0123)
  line L16 (-29.977, 43.0123) -> (-45.5655, 16.0123)
  line L17 (-45.5655, 16.0123) -> (-29.977, -10.9877)
  line L18 (-29.977, -10.9877) -> (1.1999, -10.9877)
  line L19 (-18.7187, 43.0123) -> (-23.0488, 35.5123)
  line L20 (-23.0488, 35.5123) -> (-18.7187, 28.0123)
  point P0 (-14.3886, 35.5123)
  point P1 (-14.3886, 16.0123)
  dimension "d237" = 6
  dimension "d238" = 15
  dimension "d312" = 24
  dimension "d313" = 15
  constraint coincident P0 A0.centre
  constraint parallel L0 L1
  constraint coincident P0 L0
  constraint coincident A1 L0.start
  constraint coincident A1 L0.end
  constraint tangent A1 L3
  constraint parallel L2 L3
  constraint coincident L3.start L4
  constraint coincident L3.end L5
  constraint midpoint L3 L6.start
  constraint perpendicular L3 L6
  constraint midpoint L6 P1
  constraint parallel L3 L8
  constraint coincident L3 L8.end
  constraint parallel L16 L19
  constraint tangent A1 L19
  constraint parallel L7 L20
  constraint tangent A1 L20
  constraint coincident L8 L20.end
  constraint coincident L19 L20.start
  constraint coincident L15 L19.start
  constraint coincident L19.end L20.start
  measures "d237" diameter of A0
  measures "d238" diameter of A1
  measures "d312" distance of L6.start L6.end
extrude "Extrude1''" add sketch "Sketch1" against normal blind 5 separate body contours A0 L0 picked at (-14.1661, 36.4872) makes body 20 in component "holder"
extrude "Extrude2''" add sketch "Sketch1" along normal blind 4 and the other way blind 5 contours A0 L0 picked at (-14.1661, 34.5374) bodies 20 in component "holder"
extrude "Extrude3''" add sketch "Sketch1" along normal blind 4 contours A0 A1 L0 picked at (-14.8359, 29.543) bodies 20 in component "holder"
extrude "Extrude4'''" add 1 faces at (-3.7912, 13.3886, 35.5123) along direction (0, 0, 1) blind 40 on bodies 20 bodies 20 in component "holder"
mirror "Mirror1'" about plane through (36.4957, -5.3284, 23.3879) normal (1, 0, 0) of bodies 20 makes body 21 in component "holder"
sketch "Sketch2 (3)" plane through (78.1158, 0, 0) normal (1, 0, 0) x (0, 1, 0) in component "holder"
  arc A0 (6.8886, 35.5123) -> (21.8886, 35.5123) centre (14.3886, 35.5123) ccw
  line L0 (21.8886, 35.5123) -> (21.8886, 75.5123)
  line L1 (21.8886, 75.5123) -> (6.8886, 75.5123)
  line L2 (6.8886, 75.5123) -> (6.8886, 35.5123)
  circle A1 centre (14.3886, 35.5123) radius 3.2
  point P0 (14.3886, 35.5123)
  dimension "d252" = 6.4
  constraint coincident P0 A0.centre
  measures "d252" diameter of A1
extrude "Extrude5'''" cut sketch "Sketch2 (3)" against normal up to surface (9 mm away) contours A1 bodies 21 in component "holder"
sketch "Sketch3 (4)" plane through (74.1158, 0, 0) normal (-1, 0, 0) x (0, -1, 0) in component "holder"
  circle A0 centre (-14.3886, 35.5123) radius 3.2
  arc A1 (-21.8886, 35.5123) -> (-6.8886, 35.5123) centre (-14.3886, 35.5123) ccw
  line L0 (-6.8886, 35.5123) -> (-6.8886, 75.5123)
  line L1 (-6.8886, 75.5123) -> (-21.8886, 75.5123)
  line L2 (-21.8886, 75.5123) -> (-21.8886, 35.5123)
  line L3 (-21.8886, 70.5123) -> (-6.8886, 70.5123)
  dimension "d255" = 5
  constraint coincident L2 L3.start
  constraint coincident L0 L3.end
  constraint perpendicular L0 L3
  measures "d255" distance of L1 L3
extrude "Extrude6'''" add sketch "Sketch3 (4)" along normal up to surface (75.2404 mm away) contours L0 L1 L2 L3 bodies 20 21 in component "holder"
sketch "Sketch4 (3)" plane through (0, 0, 75.5123) normal (0, 0, 1) x (-1, 0, 0) in component "holder"
  line L0 (-78.1158, -21.8886) -> (5.1245, -21.8886)
  line L1 (5.1245, -21.8886) -> (5.1245, -6.8886)
  line L2 (5.1245, -6.8886) -> (-78.1158, -6.8886)
  line L3 (-78.1158, -6.8886) -> (-78.1158, -21.8886)
  line L4 (-36.4957, -6.8886) -> (-36.4957, -21.8886) construction
  circle A0 centre (-36.4957, -14.3886) radius 3.15
  dimension "d258" = 6.3
  constraint midpoint L2 L4.start
  constraint midpoint L0 L4.end
  constraint midpoint L4 A0.centre
  measures "d258" diameter of A0
extrude "Extrude7'''" cut sketch "Sketch4 (3)" against normal up to surface (5 mm away) contours A0 bodies 20 in component "holder"
chamfer "Chamfer1'" distance 7 angle 45 2 edges at (74.1158, 14.3886, 70.5123) (-1.1245, 14.3886, 70.5123) on bodies 20 in component "holder"
fillet "Fillet1" [suppressed] in component "holder"
sketch "Sketch1 (2)" plane through (0, 0, 75.5123) normal (0, 0, 1) x (-1, 0, 0) in component "panel"
  line L0 (-78.1158, -6.8886) -> (5.1245, -6.8886)
  line L1 (5.1245, -6.8886) -> (5.1245, -21.8886)
  line L2 (5.1245, -21.8886) -> (-78.1158, -21.8886)
  line L3 (-78.1158, -21.8886) -> (-78.1158, -6.8886)
  circle A0 centre (-36.4957, -14.3886) radius 3.15
  line L4 (-78.1158, -21.8886) -> (5.1245, -21.8886)
  line L5 (5.1245, -21.8886) -> (5.1245, -6.8886)
  line L6 (5.1245, -6.8886) -> (-78.1158, -6.8886)
  line L7 (-78.1158, -6.8886) -> (-78.1158, -21.8886)
  point P0 (-36.4957, -14.3886)
  dimension "d268" = 6.3
  constraint horizontal L0
  constraint vertical L1
  constraint horizontal L2
  constraint vertical L3
  constraint coincident P0 A0.centre
  measures "d268" diameter of A0
extrude "Extrude1'''" add sketch "Sketch1 (2)" along normal blind 10 separate body contours L0 L1 L2 L3 L4 L5 L6 L7 | A0 makes body 22 in component "panel"
sketch "Sketch2 (4)" plane through (0, 0, 85.5123) normal (0, 0, 1) x (-1, 0, 0) in component "panel"
  line L0 (-78.1158, -21.8886) -> (5.1245, -21.8886)
  line L1 (5.1245, -21.8886) -> (5.1245, -6.8886)
  line L2 (5.1245, -6.8886) -> (-78.1158, -6.8886)
  line L3 (-78.1158, -6.8886) -> (-78.1158, -21.8886)
  circle A0 centre (-36.4957, -14.3886) radius 3.15
  line L4 (-48.9957, -36.0392) -> (-23.9957, -36.0392)
  line L5 (-23.9957, -36.0392) -> (-11.4957, -14.3886)
  line L6 (-11.4957, -14.3886) -> (-23.9957, 7.2621)
  line L7 (-23.9957, 7.2621) -> (-48.9957, 7.2621)
  line L8 (-48.9957, 7.2621) -> (-61.4957, -14.3886)
  line L9 (-61.4957, -14.3886) -> (-48.9957, -36.0392)
  line L10 (-41.449, -17.3086) -> (-36.4435, -20.1383)
  line L11 (-36.4435, -20.1383) -> (-31.4901, -17.2183)
  line L12 (-31.4901, -17.2183) -> (-31.5423, -11.4685)
  line L13 (-31.5423, -11.4685) -> (-36.5478, -8.6388)
  line L14 (-36.5478, -8.6388) -> (-41.5012, -11.5589)
  line L15 (-41.5012, -11.5589) -> (-41.449, -17.3086)
  point P0 (-36.4957, -14.3886)
  point P1 (-36.4957, -14.3886)
  point P2 (-36.4957, -14.3886)
  dimension "d269" = 6.3
  dimension "d270" = 25
  dimension "d271" = 5.75
  constraint coincident P2 P1
  measures "d269" diameter of A0
  measures "d270" distance of L4.start P2
  measures "d271" distance of L10.start P2
extrude "Extrude2'''" add sketch "Sketch2 (4)" against normal up to surface (10 mm away) contours L0 L4 L5 L9 | L2 L6 L7 L8 bodies 22 in component "panel"
extrude "Extrude3'''" cut sketch "Sketch2 (4)" against normal blind 6 contours A0 | L10 L11 L12 L13 L14 L15 bodies 22 in component "panel"
ref_plane "WorkPlane1" through (36.4957, 14.3886, 80.5123) normal (1, 0, 0) x (0, 1, 0) in component "panel"
sketch "Sketch3 (5)" plane through (0, 0, 75.5123) normal (0, 0, 1) x (-1, 0, 0) in component "panel"
  line L0 (-15.8258, -6.8886) -> (-15.8258, -21.8886) construction
  line L1 (5.1245, -21.8886) -> (-78.1158, -21.8886)
  line L2 (5.1245, -21.8886) -> (-15.8258, -6.8886) construction
  circle A0 centre (-5.3506, -14.3886) radius 2.5
  circle A1 centre (-5.3506, -14.3886) radius 5
  line L3 (-36.4957, 15.6927) -> (-36.4957, -44.4698)
  circle A2 centre (-67.6407, -14.3886) radius 2.5
  circle A3 centre (-67.6407, -14.3886) radius 5
  line L4 (8.0524, -14.3886) -> (1.3509, -2.7812)
  line L5 (1.3509, -2.7812) -> (-12.0521, -2.7812)
  line L6 (-12.0521, -2.7812) -> (-18.7536, -14.3886)
  line L7 (-18.7536, -14.3886) -> (-12.0521, -25.9959)
  line L8 (-12.0521, -25.9959) -> (1.3509, -25.9959)
  line L9 (1.3509, -25.9959) -> (8.0524, -14.3886)
  line L10 (-15.8258, -6.8886) -> (5.1245, -6.8886)
  line L11 (-74.3422, -2.7812) -> (-60.9392, -2.7812)
  line L12 (-81.0437, -14.3886) -> (-74.3422, -2.7812)
  line L13 (-74.3422, -25.9959) -> (-81.0437, -14.3886)
  line L14 (-60.9392, -25.9959) -> (-74.3422, -25.9959)
  line L15 (-54.2377, -14.3886) -> (-60.9392, -25.9959)
  line L16 (-60.9392, -2.7812) -> (-54.2377, -14.3886)
  point P0 (-15.8258, -6.8886)
  point P1 (-36.4957, -14.3886)
  point P2 (-5.3506, -14.3886)
  dimension "d276" = 5
  dimension "d277" = 10
  constraint coincident P0 L0.start
  constraint vertical L0
  constraint coincident L0.end L1
  constraint coincident L1.start L2.start
  constraint midpoint L2 P2
  constraint concentric A0 A1
  constraint symmetric A0 L3 A2
  constraint symmetric A1 L3 A3
  constraint coincident P2 A0.centre
  constraint parallel L5 L10
  constraint symmetric L3 L4.start L12.start
  constraint symmetric L3 L4.end L11.start
  constraint symmetric L3 L5.end L11.end
  constraint symmetric L3 L6.end L15.start
  constraint symmetric L3 L7.end L14.start
  constraint symmetric L3 L8.end L13.start
  measures "d276" diameter of A0
  measures "d277" diameter of A1
extrude "Extrude4''''" cut sketch "Sketch3 (5)" along normal up to surface (10 mm away) contours A0 | A2 bodies 22 in component "panel"
extrude "Extrude5''''" cut sketch "Sketch3 (5)" along normal blind 4 contours A1 | A3 bodies 22 in component "panel"
chamfer "Chamfer1''" distance 2.5 angle 45 2 edges at (69.9715, 13.4845, 79.5123) (7.6814, 13.4845, 79.5123) on bodies 22 in component "panel"
extrude "Extrude6''''" cut sketch "Sketch2 (4)" against normal up to surface (10 mm away) contours A0 bodies 22 in component "panel"
fillet "Fillet1'" radius 1 36 edges at (5.3506, 6.8886, 85.5123) (19.9107, -0.1867, 85.5123) (36.4957, -7.2621, 85.5123) (53.0806, -0.1867, 85.5123) (67.6407, 6.8886, 85.5123) (78.1158, 14.3886, 85.5123) (67.6407, 21.8886, 85.5123) (53.0806, 28.9639, 85.5123) (36.4957, 36.0392, 85.5123) (19.9107, 28.9639, 85.5123) (5.3506, 21.8886, 85.5123) (-5.1245, 14.3886, 85.5123) (-5.1245, 21.8886, 80.5123) (-5.1245, 6.8886, 80.5123) (15.8258, 21.8886, 80.5123) (23.9957, 36.0392, 80.5123) (48.9957, 36.0392, 80.5123) (57.1655, 21.8886, 80.5123) (78.1158, 21.8886, 80.5123) (78.1158, 6.8886, 80.5123) (57.1655, 6.8886, 80.5123) (48.9957, -7.2621, 80.5123) (23.9957, -7.2621, 80.5123) (15.8258, 6.8886, 80.5123) (-5.1245, 14.3886, 75.5123) (5.3506, 21.8886, 75.5123) (19.9107, 28.9639, 75.5123) (36.4957, 36.0392, 75.5123) (53.0806, 28.9639, 75.5123) (67.6407, 21.8886, 75.5123) (78.1158, 14.3886, 75.5123) (67.6407, 6.8886, 75.5123) (53.0806, -0.1867, 75.5123) (36.4957, -7.2621, 75.5123) (19.9107, -0.1867, 75.5123) (5.3506, 6.8886, 75.5123) on bodies 22 in component "panel"
fillet "Fillet2" radius 1 6 edges at (31.5162, 14.3434, 85.5123) (34.0451, 10.0537, 85.5123) (39.0245, 10.0988, 85.5123) (41.4751, 14.4337, 85.5123) (38.9462, 18.7235, 85.5123) (33.9668, 18.6783, 85.5123) on bodies 22 in component "panel"
chamfer "Chamfer2'" distance 3 angle 45 1 edges at (3.8755, 17.1856, 36.5971) on bodies 20 in component "holder"